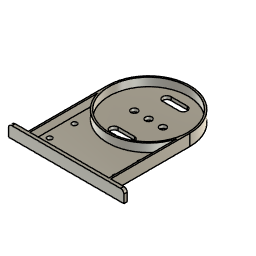
TRARM02_Link1C_50x50x7 (Autodesk Fusion 360 design; units mm, degrees)
Autodesk Fusion 360 part; units mm, degrees
note: some values were not read from the file. Set by a fixed rule: which sketch regions a step uses.
sketch "스케치1" plane through (0, 0, 0) normal (0, 0, 1) x (1, 0, 0)
  line L0 (25, 50) -> (25, 2)
  line L1 (-25, 50) -> (-25, 2)
  arc A0 (25, 50) -> (-25, 50) centre (0, 50) ccw
  line L2 (-35, 0) -> (-35, 2)
  line L3 (-35, 2) -> (-25, 2)
  line L4 (35, 0) -> (35, 2)
  line L5 (35, 2) -> (25, 2)
  line L6 (-35, 0) -> (35, 0)
  dimension "d222" = 25
  dimension "d223" = 50
  dimension "d224" = 2
  dimension "d225" = 10
  constraint vertical origin A0.centre
  constraint vertical L0
  constraint tangent L1 A0
  constraint parallel L0 L1
  constraint vertical L2
  constraint horizontal L3
  constraint vertical L4
  constraint horizontal L5
  constraint perpendicular L2 L6
  constraint equal L2 L4
  constraint equal L3 L5
  constraint tangent L0 A0
  constraint coincident origin L6
  measures "d222" radius of A0
  measures "d223" distance of origin A0.centre
  measures "d224" distance of L4.start L4.end
  measures "d225" distance of L4.end L0.end
extrude "돌출1" add sketch "스케치1" along normal blind 7
sketch "스케치24" plane through (0, 0, 7) normal (0, 0, 1) x (-1, 0, 0)
  circle A0 centre (0, -50) radius 24
  circle A1 centre (0, -50) radius 25
  line L0 (35, 0) -> (-35, 0)
  line L1 (24, -2) -> (-24, -2)
  line L2 (-24, -2) -> (-24, -43)
  line L3 (24, -2) -> (24, -43)
  line L4 (-25, -2) -> (-25, -50)
  line L5 (25, -50) -> (25, -2)
  point P0 (-25, -50)
  dimension "d226" = 48
  dimension "d227" = 1
  dimension "d228" = 1
  constraint concentric A0 A1
  constraint coincident A1 P0
  constraint parallel L0 L1
  constraint coincident A1 L2.end
  constraint perpendicular L1 L2
  constraint coincident A1 L3.end
  constraint perpendicular L1 L3
  constraint horizontal L1.end L4.start
  measures "d226" diameter of A0
  measures "d227" distance of L2 L4
  measures "d228" distance of L3 L5
extrude "돌출28" cut sketch "스케치24" against normal blind 5 contours A0 | A1 L1 L2 L3
sketch "스케치25" plane through (0, 0, 2) normal (0, 0, 1) x (-1, 0, 0)
  circle A0 centre (0, -50) radius 2
  circle A1 centre (-8.7, -50) radius 2
  circle A2 centre (8.7, -50) radius 2
  dimension "d231" = 4
  dimension "d232" = 50
  dimension "d233" = 8.7
  dimension "d234" = 8.7
  constraint equal A0 A2
  constraint equal A0 A1
  constraint horizontal A0.centre A1.centre
  constraint horizontal A0.centre A2.centre
  constraint vertical origin A0.centre
  measures "d231" diameter of A1
  measures "d232" distance of origin A0.centre
  measures "d233" distance of A0.centre A1.centre
  measures "d234" distance of A0.centre A2.centre
extrude "돌출29" cut sketch "스케치25" against normal blind 2
sketch "스케치26" plane through (0, 0, 2) normal (0, 0, 1) x (-1, 0, 0)
  circle A0 centre (-20, -25) radius 1.5
  circle A1 centre (20, -25) radius 1.5
  circle A2 centre (20, -10) radius 1.5
  circle A3 centre (-20, -10) radius 1.5
  circle A4 centre (0, -50) radius 2
  dimension "d237" = 25
  dimension "d238" = 3
  dimension "d239" = 20
  dimension "d240" = 20
  dimension "d241" = 15
  constraint equal A0 A1
  constraint horizontal A0.centre A1.centre
  constraint equal A0 A3
  constraint equal A1 A2
  constraint vertical A0.centre A3.centre
  constraint vertical A1.centre A2.centre
  constraint horizontal A2.centre A3.centre
  measures "d237" vertical distance of A0.centre A4.centre
  measures "d238" diameter of A3
  measures "d239" horizontal distance of A0.centre A4.centre
  measures "d240" horizontal distance of A1.centre A4.centre
  measures "d241" distance of A0.centre A3.centre
extrude "돌출30" cut sketch "스케치26" against normal blind 2 contours A0 | A1 | A2 | A3
fillet "필렛5" radius 2 2 edges at (-35, 1, 7) (35, 1, 7)
sketch "스케치27" plane through (0, 0, 2) normal (0, 0, 1) x (-1, 0, 0)
  circle A0 centre (0, -50) radius 2
  line L0 (5, -36.5) -> (-5, -36.5)
  line L1 (5, -31.5) -> (-5, -31.5)
  arc A1 (-5, -31.5) -> (-5, -36.5) centre (-5, -34) ccw
  arc A2 (5, -36.5) -> (5, -31.5) centre (5, -34) ccw
  line L2 (4.857, -63.5041) -> (-4.999, -63.5)
  line L3 (4.7768, -68.49) -> (-4.9974, -68.5)
  arc A3 (4.7768, -68.49) -> (4.857, -63.5041) centre (5, -66) ccw
  arc A4 (-4.999, -63.5) -> (-4.9974, -68.5) centre (-5, -66) ccw
  dimension "d247" = 5
  dimension "d248" = 10
  dimension "d249" = 5
  dimension "d254" = 16
  dimension "d256" = 16
  constraint equal A1 A2
  constraint horizontal A2.centre A1.centre
  constraint tangent L0 A1
  constraint horizontal L0
  constraint tangent L1 A1
  constraint parallel L0 L1
  constraint equal A3 A4
  constraint equal A1 A4
  constraint vertical A1.centre A4.centre
  constraint vertical A2.centre A3.centre
  constraint tangent L2 A4
  constraint tangent L3 A4
  constraint horizontal A4.centre A3.centre
  measures "d247" diameter of A1
  measures "d248" distance of A2.centre A1.centre
  measures "d249" horizontal distance of origin A1.centre
  measures "d254" vertical distance of A0.centre A1.centre
  measures "d256" vertical distance of A0.centre A4.centre
extrude "돌출31" cut sketch "스케치27" against normal blind 2 contours L0 L1 A1 A2 | L2 L3 A3 A4
